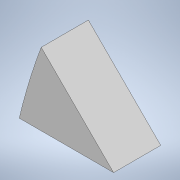
# Autodesk Inventor part: ketchenLightBracket
Saved by Autodesk Inventor 2021.2 (Build 252289000, 289)
## iProperties
Created: 2020-12-17
Part Number: ketchenLightBracket
Material: Generic
Document SubType Name: Modeling
Designer: robst
Density: 1 g/cm^3
Appearance: Default
Author: robst
Autodesk Inventor part; units mm, degrees
ref_plane "YZ Plane" through (0, 0, 0) normal (1, 0, 0) x (0, 1, 0)
ref_plane "XZ Plane" through (0, 0, 0) normal (0, 1, 0) x (-1, 0, 0)
ref_plane "XY Plane" through (0, 0, 0) normal (0, 0, 1) x (1, 0, 0)
sketch "Sketch1" plane through (0, 0, 0) normal (0, 0, 1) x (1, 0, 0)
  line L0 (0, 0) -> (0, 304.8) construction
  arc A0 (0, 304.8) -> (0, 0) centre (292.9271, 152.4) ccw
  line L1 (0, 152.4) -> (-37.2729, 152.4) construction
  line L2 (-28.3603, 228.6) -> (22.4397, 228.6)
  line L3 (22.4397, 228.6) -> (-16.5351, 267.5747)
  line L4 (-28.3603, 228.6) -> (22.4397, 228.6)
  dimension "d0" = 304.8
  dimension "d1" = 330.2
  dimension "d2" = 50.8
  dimension "d3" = 45
  dimension "d4" = 76.2
  constraints: 10 end point, 5 point on circle, 1 centre point, 1 collinear, 1 horizontal, 1 midpoint, 1 vertical
  measures "d0" distance of L0.end L0.start
  measures "d1" radius of A0
  measures "d2" distance of L2.start L2.end
  measures "d3" angle of L3 L2
  measures "d4" distance between parallel lines of L2 L1
extrude "Extrusion1" add sketch "Sketch1" along normal mid plane 25.4
body "Solid1"
